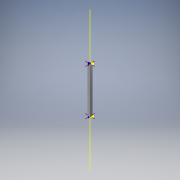
# Autodesk Inventor part: Pins
Saved by Autodesk Inventor 2019 (Build 230136000, 136)
## iProperties
Created: 2019-03-11
Part Number: Pins
Material: Aluminium 6061
Document SubType Name: Blech
Designer: manue
Density: 2.7 g/cm^3
Sheet Metal Rule: Standard_mm
Appearance: Aluminium - poliert
Author: manue
Autodesk Inventor part; units mm, degrees
ref_plane "YZ Plane" through (0, 0, 0) normal (1, 0, 0) x (0, 1, 0)
ref_plane "XZ Plane" through (0, 0, 0) normal (0, 1, 0) x (-1, 0, 0)
ref_plane "XY Plane" through (0, 0, 0) normal (0, 0, 1) x (1, 0, 0)
sketch "Skizze1" plane through (0, 0, 0) normal (0, 0, 1) x (1, 0, 0)
  line L0 (0, 0) -> (-0.6, 0)
  line L1 (-0.6, 0) -> (-0.6, -10.7)
  line L2 (-0.6, -10.7) -> (0, -10.7)
  line L3 (0, -10.7) -> (0, 0)
  dimension "d0" = 0.6
  dimension "d1" = 10.7
  measures "d0" distance of L2.end L1.end
  measures "d1" distance of L1.end L0.end
extrude "Grobblech1" add sketch "Skizze1" along normal blind 0.6
chamfer "Fase1" distance 0.1 angle 45 8 edges at (-0.6, -10.7, 0.3) (-0.3, -10.7, 0) (0, -10.7, 0.3) (-0.3, -10.7, 0.6) (-0.3, 0, 0) (-0.6, 0, 0.3) (-0.3, 0, 0.6) (0, 0, 0.3)
sketch "Skizze2" plane through (-0.5, -10.7, 0.1) normal (0, -1, 0) x (1, 0, 0)
  line L0 (0.4, 0) -> (0, 0) projected
  line L1 (0.4, 0.4) -> (0.4, 0) projected
  line L2 (0, 0.4) -> (0.4, 0.4) projected
  line L3 (0, 0) -> (0, 0.4) projected
  point P0 (0.5, -0.1)
  point P1 (0.2, 0.2)
  point P2 (0, 0.2)
  point P3 (0.2, 0.4)
  constraints: 2 midpoint, 1 horizontal alignment, 1 vertical alignment
sketch "Skizze3" plane through (-0.5, 0, 0.1) normal (0, 1, 0) x (1, 0, 0)
  line L0 (0, 0) -> (0.4, 0) construction
  line L1 (0, -0.4) -> (0, 0) construction
  line L2 (0.4, -0.4) -> (0, -0.4) construction
  line L3 (0.4, 0) -> (0.4, -0.4) construction
  point P0 (0.5, 0.1)
  point P1 (0.2, -0.2)
  point P2 (0, -0.2)
  point P3 (0.2, -0.4)
  constraints: 2 midpoint, 1 horizontal alignment, 1 vertical alignment
equation "\"d2\" = Stärke"
equation "\"Biegeradius\" = Stärke"
equation "\"BreiteBiegungsfreistellung\" = Stärke"
equation "\"TiefeBiegungsfreistellung\" = 0.5 * Stärke"
equation "\"GrößeEckenfreistellung\" = 4 * Stärke"
equation "\"MinimalRest\" = 2 * Stärke"
equation "\"Übergangsradius\" = Biegeradius"
equation "\"JacobiRadiusGröße\" = Biegeradius"
equation "\"Abstandsgröße\" = Stärke"
equation "\"Stärke\" = 0.6"
